Autodesk Fusion 360 part; units mm, degrees
note: some values were not read from the file. Set by a fixed rule: which sketch regions a step uses.
(part 52 of 59)
  spline S32 degree 5 poles (-9.8472, -14.8251) (-9.8472, -14.8252) (-9.8473, -14.8254) (-9.8474, -14.8257) (-9.8475, -14.8262) (-9.8478, -14.8269) (-9.8481, -14.8277) (-9.8484, -14.8286) (-9.8487, -14.8296) (-9.8491, -14.8308) (-9.8495, -14.832) (-9.85, -14.8334) (-9.8505, -14.8348) (-9.851, -14.8364) (-9.8515, -14.838) (-9.8521, -14.8398) (-9.8527, -14.8416) (-9.8533, -14.8435) (-9.8539, -14.8456) (-9.8546, -14.8477) (-9.8553, -14.8499) (-9.856, -14.8523) (-9.8568, -14.8547) (-9.8575, -14.8572) (-9.8583, -14.8598) (-9.8591, -14.8625) (-9.86, -14.8652) (-9.8608, -14.8681) (-9.8617, -14.871) (-9.8626, -14.8741) (-9.8635, -14.8772) (-9.8645, -14.8804) (-9.8654, -14.8837) (-9.8664, -14.887) (-9.8674, -14.8905) (-9.8684, -14.894) (-9.8694, -14.8976) (-9.8704, -14.9013) (-9.8715, -14.9051) (-9.8725, -14.909) (-9.8736, -14.9129) (-9.8747, -14.9169) (-9.8758, -14.921) (-9.8769, -14.9252) (-9.878, -14.9294) (-9.8792, -14.9337) (-9.8803, -14.9381) (-9.8815, -14.9426) (-9.8827, -14.9471) (-9.8838, -14.9517) (-9.885, -14.9564) (-9.8862, -14.9612) (-9.8874, -14.966) (-9.8887, -14.9709) (-9.8899, -14.9759) (-9.8911, -14.981) (-9.8924, -14.9861) (-9.8936, -14.9912) (-9.8949, -14.9965) (-9.8962, -15.0018) (-9.8974, -15.0072) (-9.8987, -15.0127) (-9.9, -15.0182) (-9.9013, -15.0238) (-9.9026, -15.0294) (-9.9039, -15.0352) (-9.9052, -15.0409) (-9.9065, -15.0468) (-9.9079, -15.0527) (-9.9092, -15.0587) (-9.9105, -15.0647) (-9.9118, -15.0709) (-9.9132, -15.077) (-9.9145, -15.0833) (-9.9158, -15.0896) (-9.9172, -15.0959) (-9.9185, -15.1023) (-9.9199, -15.1088) (-9.9212, -15.1154) (-9.9225, -15.122) (-9.9239, -15.1286) (-9.9252, -15.1353) (-9.9266, -15.1421) (-9.9279, -15.149) (-9.9293, -15.1559) (-9.9306, -15.1628) (-9.932, -15.1698) (-9.9333, -15.1769) (-9.9347, -15.1841) (-9.936, -15.1912) (-9.9374, -15.1985) (-9.9387, -15.2058) (-9.9401, -15.2132) (-9.9414, -15.2206) (-9.9428, -15.228) (-9.9441, -15.2356) (-9.9454, -15.2431) (-9.9468, -15.2508) (-9.9481, -15.2585) (-9.9494, -15.2662) (-9.9508, -15.274) (-9.9521, -15.2819) (-9.9534, -15.2898) (-9.9547, -15.2977) (-9.956, -15.3057) (-9.9573, -15.3138) (-9.9586, -15.3219) (-9.9599, -15.3301) (-9.9612, -15.3383) (-9.9625, -15.3466) (-9.9638, -15.3549) (-9.9651, -15.3633) (-9.9664, -15.3717) (-9.9676, -15.3802) (-9.9689, -15.3887) (-9.9701, -15.3973) (-9.9714, -15.4059) (-9.9726, -15.4146) (-9.9739, -15.4233) (-9.9751, -15.4321) (-9.9763, -15.4409) (-9.9776, -15.4498) (-9.9788, -15.4587) (-9.98, -15.4677) (-9.9812, -15.4767) (-9.9824, -15.4858) (-9.9836, -15.4949) (-9.9847, -15.504) (-9.9859, -15.5133) (-9.9871, -15.5225) (-9.9882, -15.5318) (-9.9894, -15.5412) (-9.9905, -15.5506) (-9.9916, -15.56) (-9.9928, -15.5695) (-9.9939, -15.579) (-9.995, -15.5886) (-9.9961, -15.5982) (-9.9972, -15.6079) (-9.9983, -15.6176) (-9.9993, -15.6274) (-10.0004, -15.6372) (-10.0014, -15.647) (-10.0025, -15.6569) (-10.0035, -15.6668) (-10.0045, -15.6768) (-10.0055, -15.6868) (-10.0065, -15.6969) (-10.0075, -15.707) (-10.0085, -15.7172) (-10.0095, -15.7274) (-10.0104, -15.7376) (-10.0114, -15.7479) (-10.0123, -15.7582) (-10.0133, -15.7686) (-10.0142, -15.779) (-10.0151, -15.7894) (-10.016, -15.7999) (-10.0169, -15.8105) (-10.0177, -15.821) (-10.0186, -15.8317) (-10.0195, -15.8423) (-10.0203, -15.853) (-10.0211, -15.8638) (-10.0219, -15.8745) (-10.0227, -15.8854) (-10.0235, -15.8962) (-10.0243, -15.9071) (-10.0251, -15.9181) (-10.0258, -15.929) (-10.0266, -15.94) (-10.0273, -15.9511) (-10.028, -15.9622) (-10.0287, -15.9733) (-10.0294, -15.9845) (-10.0301, -15.9957) (-10.0308, -16.007) (-10.0314, -16.0183) (-10.0321, -16.0296) (-10.0327, -16.041) (-10.0333, -16.0524) (-10.0339, -16.0638) (-10.0345, -16.0753) (-10.0351, -16.0868) (-10.0356, -16.0984) (-10.0362, -16.11) (-10.0367, -16.1216) (-10.0372, -16.1333) (-10.0377, -16.145) (-10.0382, -16.1567) (-10.0387, -16.1685) (-10.0392, -16.1803) (-10.0396, -16.1922) (-10.04, -16.2041) (-10.0405, -16.216) (-10.0409, -16.228) (-10.0412, -16.24) (-10.0416, -16.252) (-10.042, -16.2641) (-10.0423, -16.2762) (-10.0427, -16.2883) (-10.043, -16.3005) (-10.0433, -16.3127) (-10.0436, -16.3249) (-10.0438, -16.3372) (-10.0441, -16.3495) (-10.0443, -16.3619) (-10.0445, -16.3743) (-10.0448, -16.3867) (-10.0449, -16.3991) (-10.0451, -16.4116) (-10.0453, -16.4241) (-10.0454, -16.4367) (-10.0456, -16.4493) (-10.0457, -16.4619) (-10.0458, -16.4745) (-10.0458, -16.4872) (-10.0459, -16.5) (-10.046, -16.5127) (-10.046, -16.5255) (-10.046, -16.5383) (-10.046, -16.5512) (-10.046, -16.5641) (-10.046, -16.577) (-10.0459, -16.5899) (-10.0458, -16.6029) (-10.0458, -16.6159) (-10.0457, -16.629) (-10.0455, -16.642) (-10.0454, -16.6551) (-10.0453, -16.6683) (-10.0451, -16.6815) (-10.0449, -16.6947) (-10.0447, -16.7079) (-10.0445, -16.7212) (-10.0442, -16.7345) (-10.044, -16.7478) (-10.0437, -16.7612) (-10.0434, -16.7745) (-10.0431, -16.788) (-10.0428, -16.8014) (-10.0425, -16.8122) (-10.0423, -16.8203) (-10.0422, -16.8257) (-10.0421, -16.8284) knots 0 0 0 0 0 0 0.00416667 0.00833333 0.0125 0.01666667 0.02083333 0.025 0.02916667 0.03333333 0.0375 0.04166667 0.04583333 0.05 0.05416667 0.05833333 0.0625 0.06666667 0.07083333 0.075 0.07916667 0.08333333 0.0875 0.09166667 0.09583333 0.1 0.10416667 0.10833333 0.1125 0.11666667 0.12083333 0.125 0.12916667 0.13333333 0.1375 0.14166667 0.14583333 0.15 0.15416667 0.15833333 0.1625 0.16666667 0.17083333 0.175 0.17916667 0.18333333 0.1875 0.19166667 0.19583333 0.2 0.20416667 0.20833333 0.2125 0.21666667 0.22083333 0.225 0.22916667 0.23333333 0.2375 0.24166667 0.24583333 0.25 0.25416667 0.25833333 0.2625 0.26666667 0.27083333 0.275 0.27916667 0.28333333 0.2875 0.29166667 0.29583333 0.3 0.30416667 0.30833333 0.3125 0.31666667 0.32083333 0.325 0.32916667 0.33333333 0.3375 0.34166667 0.34583333 0.35 0.35416667 0.35833333 0.3625 0.36666667 0.37083333 0.375 0.37916667 0.38333333 0.3875 0.39166667 0.39583333 0.4 0.40416667 0.40833333 0.4125 0.41666667 0.42083333 0.425 0.42916667 0.43333333 0.4375 0.44166667 0.44583333 0.45 0.45416667 0.45833333 0.4625 0.46666667 0.47083333 0.475 0.47916667 0.48333333 0.4875 0.49166667 0.49583333 0.5 0.50416667 0.50833333 0.5125 0.51666667 0.52083333 0.525 0.52916667 0.53333333 0.5375 0.54166667 0.54583333 0.55 0.55416667 0.55833333 0.5625 0.56666667 0.57083333 0.575 0.57916667 0.58333333 0.5875 0.59166667 0.59583333 0.6 0.60416667 0.60833333 0.6125 0.61666667 0.62083333 0.625 0.62916667 0.63333333 0.6375 0.64166667 0.64583333 0.65 0.65416667 0.65833333 0.6625 0.66666667 0.67083333 0.675 0.67916667 0.68333333 0.6875 0.69166667 0.69583333 0.7 0.70416667 0.70833333 0.7125 0.71666667 0.72083333 0.725 0.72916667 0.73333333 0.7375 0.74166667 0.74583333 0.75 0.75416667 0.75833333 0.7625 0.76666667 0.77083333 0.775 0.77916667 0.78333333 0.7875 0.79166667 0.79583333 0.8 0.80416667 0.80833333 0.8125 0.81666667 0.82083333 0.825 0.82916667 0.83333333 0.8375 0.84166667 0.84583333 0.85 0.85416667 0.85833333 0.8625 0.86666667 0.87083333 0.875 0.87916667 0.88333333 0.8875 0.89166667 0.89583333 0.9 0.90416667 0.90833333 0.9125 0.91666667 0.92083333 0.925 0.92916667 0.93333333 0.9375 0.94166667 0.94583333 0.95 0.95416667 0.95833333 0.9625 0.96666667 0.97083333 0.975 0.97916667 0.98333333 0.9875 0.99166667 0.99583333 1 1 1 1 1 1
  arc A33 (-10.0421, -16.8284) -> (-9.1146, -17.1298) centre (0, 12.5) ccw
  spline S33 degree 5 poles (-9.1146, -17.1298) (-9.1129, -17.1276) (-9.1096, -17.1234) (-9.1047, -17.1169) (-9.0981, -17.1084) (-9.09, -17.0977) (-9.0818, -17.087) (-9.0737, -17.0763) (-9.0657, -17.0657) (-9.0576, -17.055) (-9.0496, -17.0444) (-9.0416, -17.0338) (-9.0337, -17.0232) (-9.0258, -17.0127) (-9.0179, -17.0021) (-9.0101, -16.9915) (-9.0022, -16.981) (-8.9945, -16.9705) (-8.9867, -16.96) (-8.979, -16.9495) (-8.9713, -16.9391) (-8.9637, -16.9286) (-8.956, -16.9182) (-8.9485, -16.9078) (-8.9409, -16.8974) (-8.9334, -16.887) (-8.9259, -16.8766) (-8.9184, -16.8663) (-8.911, -16.856) (-8.9036, -16.8457) (-8.8963, -16.8354) (-8.8889, -16.8251) (-8.8816, -16.8148) (-8.8744, -16.8046) (-8.8671, -16.7944) (-8.86, -16.7842) (-8.8528, -16.774) (-8.8457, -16.7638) (-8.8386, -16.7537) (-8.8315, -16.7435) (-8.8245, -16.7334) (-8.8175, -16.7233) (-8.8105, -16.7132) (-8.8036, -16.7032) (-8.7967, -16.6932) (-8.7898, -16.6831) (-8.783, -16.6731) (-8.7762, -16.6632) (-8.7694, -16.6532) (-8.7626, -16.6433) (-8.7559, -16.6334) (-8.7493, -16.6235) (-8.7426, -16.6136) (-8.736, -16.6037) (-8.7295, -16.5939) (-8.7229, -16.5841) (-8.7164, -16.5743) (-8.7099, -16.5646) (-8.7035, -16.5548) (-8.6971, -16.5451) (-8.6907, -16.5354) (-8.6844, -16.5257) (-8.6781, -16.516) (-8.6718, -16.5064) (-8.6656, -16.4968) (-8.6593, -16.4872) (-8.6532, -16.4776) (-8.647, -16.4681) (-8.6409, -16.4586) (-8.6348, -16.4491) (-8.6288, -16.4396) (-8.6228, -16.4302) (-8.6168, -16.4207) (-8.6109, -16.4113) (-8.605, -16.402) (-8.5991, -16.3926) (-8.5932, -16.3833) (-8.5874, -16.374) (-8.5817, -16.3647) (-8.5759, -16.3555) (-8.5702, -16.3462) (-8.5645, -16.337) (-8.5589, -16.3279) (-8.5533, -16.3187) (-8.5477, -16.3096) (-8.5422, -16.3005) (-8.5367, -16.2914) (-8.5312, -16.2824) (-8.5257, -16.2734) (-8.5203, -16.2644) (-8.515, -16.2554) (-8.5096, -16.2465) (-8.5043, -16.2376) (-8.499, -16.2287) (-8.4938, -16.2199) (-8.4886, -16.211) (-8.4834, -16.2022) (-8.4783, -16.1935) (-8.4732, -16.1847) (-8.4681, -16.176) (-8.463, -16.1674) (-8.458, -16.1587) (-8.4531, -16.1501) (-8.4481, -16.1415) (-8.4432, -16.133) (-8.4384, -16.1244) (-8.4335, -16.116) (-8.4287, -16.1075) (-8.4239, -16.0991) (-8.4192, -16.0907) (-8.4145, -16.0823) (-8.4098, -16.074) (-8.4052, -16.0657) (-8.4006, -16.0574) (-8.396, -16.0491) (-8.3915, -16.0409) (-8.387, -16.0328) (-8.3825, -16.0246) (-8.3781, -16.0165) (-8.3737, -16.0085) (-8.3693, -16.0004) (-8.365, -15.9924) (-8.3607, -15.9845) (-8.3565, -15.9765) (-8.3522, -15.9686) (-8.348, -15.9608) (-8.3439, -15.9529) (-8.3398, -15.9452) (-8.3357, -15.9374) (-8.3316, -15.9297) (-8.3276, -15.922) (-8.3236, -15.9144) (-8.3196, -15.9068) (-8.3157, -15.8992) (-8.3118, -15.8917) (-8.308, -15.8842) (-8.3042, -15.8767) (-8.3004, -15.8693) (-8.2966, -15.8619) (-8.2929, -15.8546) (-8.2892, -15.8473) (-8.2856, -15.8401) (-8.282, -15.8329) (-8.2784, -15.8257) (-8.2748, -15.8186) (-8.2713, -15.8115) (-8.2678, -15.8044) (-8.2644, -15.7974) (-8.261, -15.7905) (-8.2576, -15.7835) (-8.2543, -15.7767) (-8.251, -15.7698) (-8.2477, -15.763) (-8.2445, -15.7563) (-8.2412, -15.7496) (-8.2381, -15.7429) (-8.2349, -15.7363) (-8.2318, -15.7298) (-8.2288, -15.7233) (-8.2257, -15.7168) (-8.2227, -15.7104) (-8.2198, -15.704) (-8.2169, -15.6977) (-8.214, -15.6914) (-8.2111, -15.6851) (-8.2083, -15.679) (-8.2055, -15.6728) (-8.2027, -15.6667) (-8.2, -15.6607) (-8.1973, -15.6547) (-8.1947, -15.6488) (-8.192, -15.6429) (-8.1895, -15.6371) (-8.1869, -15.6313) (-8.1844, -15.6256) (-8.1819, -15.6199) (-8.1795, -15.6143) (-8.177, -15.6087) (-8.1747, -15.6032) (-8.1723, -15.5978) (-8.17, -15.5924) (-8.1677, -15.587) (-8.1655, -15.5818) (-8.1633, -15.5765) (-8.1611, -15.5714) (-8.159, -15.5663) (-8.1569, -15.5612) (-8.1548, -15.5562) (-8.1528, -15.5513) (-8.1508, -15.5464) (-8.1488, -15.5416) (-8.1469, -15.5369) (-8.145, -15.5322) (-8.1432, -15.5276) (-8.1413, -15.523) (-8.1395, -15.5185) (-8.1378, -15.5141) (-8.1361, -15.5097) (-8.1344, -15.5054) (-8.1327, -15.5012) (-8.1311, -15.497) (-8.1295, -15.4929) (-8.128, -15.4889) (-8.1265, -15.4849) (-8.125, -15.4811) (-8.1236, -15.4772) (-8.1222, -15.4735) (-8.1208, -15.4698) (-8.1194, -15.4662) (-8.1181, -15.4627) (-8.1169, -15.4593) (-8.1156, -15.4559) (-8.1144, -15.4526) (-8.1133, -15.4494) (-8.1121, -15.4462) (-8.1111, -15.4432) (-8.11, -15.4402) (-8.109, -15.4373) (-8.108, -15.4345) (-8.107, -15.4318) (-8.1061, -15.4291) (-8.1052, -15.4265) (-8.1044, -15.4241) (-8.1036, -15.4217) (-8.1028, -15.4194) (-8.102, -15.4172) (-8.1013, -15.415) (-8.1007, -15.413) (-8.1, -15.4111) (-8.0994, -15.4092) (-8.0988, -15.4075) (-8.0983, -15.4058) (-8.0978, -15.4043) (-8.0973, -15.4028) (-8.0969, -15.4015) (-8.0965, -15.4002) (-8.0962, -15.3991) (-8.0958, -15.398) (-8.0956, -15.3971) (-8.0953, -15.3963) (-8.0951, -15.3956) (-8.0949, -15.3951) (-8.0948, -15.3948) (-8.0948, -15.3946) (-8.0948, -15.3945) knots -1 -1 -1 -1 -1 -1 -0.99583333 -0.99166667 -0.9875 -0.98333333 -0.97916667 -0.975 -0.97083333 -0.96666667 -0.9625 -0.95833333 -0.95416667 -0.95 -0.94583333 -0.94166667 -0.9375 -0.93333333 -0.92916667 -0.925 -0.92083333 -0.91666667 -0.9125 -0.90833333 -0.90416667 -0.9 -0.89583333 -0.89166667 -0.8875 -0.88333333 -0.87916667 -0.875 -0.87083333 -0.86666667 -0.8625 -0.85833333 -0.85416667 -0.85 -0.84583333 -0.84166667 -0.8375 -0.83333333 -0.82916667 -0.825 -0.82083333 -0.81666667 -0.8125 -0.80833333 -0.80416667 -0.8 -0.79583333 -0.79166667 -0.7875 -0.78333333 -0.77916667 -0.775 -0.77083333 -0.76666667 -0.7625 -0.75833333 -0.75416667 -0.75 -0.74583333 -0.74166667 -0.7375 -0.73333333 -0.72916667 -0.725 -0.72083333 -0.71666667 -0.7125 -0.70833333 -0.70416667 -0.7 -0.69583333 -0.69166667 -0.6875 -0.68333333 -0.67916667 -0.675 -0.67083333 -0.66666667 -0.6625 -0.65833333 -0.65416667 -0.65 -0.64583333 -0.64166667 -0.6375 -0.63333333 -0.62916667 -0.625 -0.62083333 -0.61666667 -0.6125 -0.60833333 -0.60416667 -0.6 -0.59583333 -0.59166667 -0.5875 -0.58333333 -0.57916667 -0.575 -0.57083333 -0.56666667 -0.5625 -0.55833333 -0.55416667 -0.55 -0.54583333 -0.54166667 -0.5375 -0.53333333 -0.52916667 -0.525 -0.52083333 -0.51666667 -0.5125 -0.50833333 -0.50416667 -0.5 -0.49583333 -0.49166667 -0.4875 -0.48333333 -0.47916667 -0.475 -0.47083333 -0.46666667 -0.4625 -0.45833333 -0.45416667 -0.45 -0.44583333 -0.44166667 -0.4375 -0.43333333 -0.42916667 -0.425 -0.42083333 -0.41666667 -0.4125 -0.40833333 -0.40416667 -0.4 -0.39583333 -0.39166667 -0.3875 -0.38333333 -0.37916667 -0.375 -0.37083333 -0.36666667 -0.3625 -0.35833333 -0.35416667 -0.35 -0.34583333 -0.34166667 -0.3375 -0.33333333 -0.32916667 -0.325 -0.32083333 -0.31666667 -0.3125 -0.30833333 -0.30416667 -0.3 -0.29583333 -0.29166667 -0.2875 -0.28333333 -0.27916667 -0.275 -0.27083333 -0.26666667 -0.2625 -0.25833333 -0.25416667 -0.25 -0.24583333 -0.24166667 -0.2375 -0.23333333 -0.22916667 -0.225 -0.22083333 -0.21666667 -0.2125 -0.20833333 -0.20416667 -0.2 -0.19583333 -0.19166667 -0.1875 -0.18333333 -0.17916667 -0.175 -0.17083333 -0.16666667 -0.1625 -0.15833333 -0.15416667 -0.15 -0.14583333 -0.14166667 -0.1375 -0.13333333 -0.12916667 -0.125 -0.12083333 -0.11666667 -0.1125 -0.10833333 -0.10416667 -0.1 -0.09583333 -0.09166667 -0.0875 -0.08333333 -0.07916667 -0.075 -0.07083333 -0.06666667 -0.0625 -0.05833333 -0.05416667 -0.05 -0.04583333 -0.04166667 -0.0375 -0.03333333 -0.02916667 -0.025 -0.02083333 -0.01666667 -0.0125 -0.00833333 -0.00416667 0 0 0 0 0 0
  line L67 (-8.0948, -15.3945) -> (-8.0945, -15.3937)
  line L68 (-8.0945, -15.3937) -> (-8.0125, -15.1109)
  arc A34 (-8.0125, -15.1109) -> (-6.8665, -15.418) centre (0, 12.5) ccw
  line L69 (-6.8665, -15.418) -> (-6.9368, -15.7039)
  line L70 (-6.9368, -15.7039) -> (-6.937, -15.7047)
  spline S34 degree 5 poles (-6.937, -15.7047) (-6.937, -15.7048) (-6.937, -15.705) (-6.9371, -15.7053) (-6.9372, -15.7058) (-6.9374, -15.7065) (-6.9376, -15.7074) (-6.9378, -15.7083) (-6.9381, -15.7094) (-6.9383, -15.7106) (-6.9386, -15.7118) (-6.9389, -15.7132) (-6.9392, -15.7147) (-6.9396, -15.7163) (-6.9399, -15.718) (-6.9403, -15.7198) (-6.9407, -15.7217) (-6.9411, -15.7237) (-6.9416, -15.7258) (-6.942, -15.728) (-6.9425, -15.7303) (-6.9429, -15.7327) (-6.9434, -15.7351) (-6.9439, -15.7377) (-6.9445, -15.7404) (-6.945, -15.7431) (-6.9455, -15.746) (-6.9461, -15.7489) (-6.9466, -15.7519) (-6.9472, -15.755) (-6.9478, -15.7582) (-6.9484, -15.7615) (-6.949, -15.7649) (-6.9496, -15.7683) (-6.9502, -15.7719) (-6.9508, -15.7755) (-6.9515, -15.7792) (-6.9521, -15.783) (-6.9528, -15.7868) (-6.9534, -15.7908) (-6.9541, -15.7948) (-6.9547, -15.7989) (-6.9554, -15.8031) (-6.9561, -15.8074) (-6.9568, -15.8117) (-6.9574, -15.8161) (-6.9581, -15.8206) (-6.9588, -15.8252) (-6.9595, -15.8298) (-6.9602, -15.8345) (-6.9609, -15.8393) (-6.9616, -15.8442) (-6.9623, -15.8491) (-6.963, -15.8541) (-6.9637, -15.8592) (-6.9644, -15.8643) (-6.9651, -15.8695) (-6.9658, -15.8748) (-6.9665, -15.8802) (-6.9672, -15.8856) (-6.9679, -15.8911) (-6.9686, -15.8966) (-6.9693, -15.9023) (-6.97, -15.908) (-6.9707, -15.9137) (-6.9714, -15.9196) (-6.9721, -15.9255) (-6.9728, -15.9314) (-6.9735, -15.9374) (-6.9742, -15.9435) (-6.9749, -15.9497) (-6.9756, -15.9559) (-6.9763, -15.9622) (-6.9769, -15.9685) (-6.9776, -15.9749) (-6.9783, -15.9814) (-6.9789, -15.9879) (-6.9796, -15.9945) (-6.9803, -16.0011) (-6.9809, -16.0078) (-6.9816, -16.0146) (-6.9822, -16.0214) (-6.9828, -16.0283) (-6.9835, -16.0353) (-6.9841, -16.0423) (-6.9847, -16.0493) (-6.9853, -16.0564) (-6.9859, -16.0636) (-6.9865, -16.0709) (-6.9871, -16.0781) (-6.9877, -16.0855) (-6.9882, -16.0929) (-6.9888, -16.1004) (-6.9894, -16.1079) (-6.9899, -16.1154) (-6.9905, -16.1231) (-6.991, -16.1307) (-6.9915, -16.1385) (-6.9921, -16.1463) (-6.9926, -16.1541) (-6.9931, -16.162) (-6.9936, -16.17) (-6.994, -16.178) (-6.9945, -16.186) (-6.995, -16.1941) (-6.9954, -16.2023) (-6.9959, -16.2105) (-6.9963, -16.2187) (-6.9968, -16.227) (-6.9972, -16.2354) (-6.9976, -16.2438) (-6.998, -16.2523) (-6.9984, -16.2608) (-6.9987, -16.2694) (-6.9991, -16.278) (-6.9995, -16.2866) (-6.9998, -16.2953) (-7.0001, -16.3041) (-7.0005, -16.3129) (-7.0008, -16.3218) (-7.0011, -16.3307) (-7.0014, -16.3396) (-7.0016, -16.3486) (-7.0019, -16.3577) (-7.0021, -16.3668) (-7.0024, -16.3759) (-7.0026, -16.3851) (-7.0028, -16.3943) (-7.003, -16.4036) (-7.0032, -16.4129) (-7.0034, -16.4223) (-7.0036, -16.4317) (-7.0037, -16.4412) (-7.0038, -16.4507) (-7.004, -16.4602) (-7.0041, -16.4698) (-7.0042, -16.4795) (-7.0043, -16.4892) (-7.0043, -16.4989) (-7.0044, -16.5087) (-7.0044, -16.5185) (-7.0045, -16.5284) (-7.0045, -16.5383) (-7.0045, -16.5482) (-7.0045, -16.5582) (-7.0044, -16.5682) (-7.0044, -16.5783) (-7.0043, -16.5884) (-7.0043, -16.5986) (-7.0042, -16.6088) (-7.0041, -16.619) (-7.004, -16.6293) (-7.0038, -16.6396) (-7.0037, -16.65) (-7.0035, -16.6604) (-7.0034, -16.6708) (-7.0032, -16.6813) (-7.003, -16.6919) (-7.0028, -16.7024) (-7.0025, -16.713) (-7.0023, -16.7237) (-7.002, -16.7344) (-7.0017, -16.7451) (-7.0014, -16.7559) (-7.0011, -16.7667) (-7.0008, -16.7775) (-7.0004, -16.7884) (-7.0001, -16.7993) (-6.9997, -16.8103) (-6.9993, -16.8213) (-6.9989, -16.8323) (-6.9984, -16.8434) (-6.998, -16.8545) (-6.9975, -16.8657) (-6.997, -16.8768) (-6.9965, -16.8881) (-6.996, -16.8993) (-6.9955, -16.9106) (-6.995, -16.922) (-6.9944, -16.9333) (-6.9938, -16.9447) (-6.9932, -16.9562) (-6.9926, -16.9677) (-6.992, -16.9792) (-6.9913, -16.9907) (-6.9906, -17.0023) (-6.99, -17.014) (-6.9892, -17.0256) (-6.9885, -17.0373) (-6.9878, -17.049) (-6.987, -17.0608) (-6.9863, -17.0726) (-6.9855, -17.0844) (-6.9846, -17.0963) (-6.9838, -17.1082) (-6.983, -17.1201) (-6.9821, -17.1321) (-6.9812, -17.1441) (-6.9803, -17.1562) (-6.9794, -17.1682) (-6.9784, -17.1803) (-6.9775, -17.1925) (-6.9765, -17.2047) (-6.9755, -17.2169) (-6.9745, -17.2291) (-6.9735, -17.2414) (-6.9724, -17.2537) (-6.9713, -17.266) (-6.9702, -17.2784) (-6.9691, -17.2908) (-6.968, -17.3032) (-6.9669, -17.3157) (-6.9657, -17.3282) (-6.9645, -17.3407) (-6.9633, -17.3533) (-6.9621, -17.3659) (-6.9608, -17.3785) (-6.9596, -17.3912) (-6.9583, -17.4039) (-6.957, -17.4166) (-6.9556, -17.4293) (-6.9543, -17.4421) (-6.9529, -17.4549) (-6.9516, -17.4678) (-6.9501, -17.4806) (-6.9487, -17.4935) (-6.9473, -17.5065) (-6.9458, -17.5194) (-6.9443, -17.5324) (-6.9428, -17.5455) (-6.9413, -17.5585) (-6.9398, -17.5716) (-6.9382, -17.5847) (-6.9366, -17.5979) (-6.935, -17.611) (-6.9334, -17.6242) (-6.9317, -17.6375) (-6.9301, -17.6507) (-6.9284, -17.664) (-6.9267, -17.6773) (-6.925, -17.6907) (-6.9236, -17.7014) (-6.9225, -17.7094) (-6.9218, -17.7148) (-6.9214, -17.7174) knots 0 0 0 0 0 0 0.00416667 0.00833333 0.0125 0.01666667 0.02083333 0.025 0.02916667 0.03333333 0.0375 0.04166667 0.04583333 0.05 0.05416667 0.05833333 0.0625 0.06666667 0.07083333 0.075 0.07916667 0.08333333 0.0875 0.09166667 0.09583333 0.1 0.10416667 0.10833333 0.1125 0.11666667 0.12083333 0.125 0.12916667 0.13333333 0.1375 0.14166667 0.14583333 0.15 0.15416667 0.15833333 0.1625 0.16666667 0.17083333 0.175 0.17916667 0.18333333 0.1875 0.19166667 0.19583333 0.2 0.20416667 0.20833333 0.2125 0.21666667 0.22083333 0.225 0.22916667 0.23333333 0.2375 0.24166667 0.24583333 0.25 0.25416667 0.25833333 0.2625 0.26666667 0.27083333 0.275 0.27916667 0.28333333 0.2875 0.29166667 0.29583333 0.3 0.30416667 0.30833333 0.3125 0.31666667 0.32083333 0.325 0.32916667 0.33333333 0.3375 0.34166667 0.34583333 0.35 0.35416667 0.35833333 0.3625 0.36666667 0.37083333 0.375 0.37916667 0.38333333 0.3875 0.39166667 0.39583333 0.4 0.40416667 0.40833333 0.4125 0.41666667 0.42083333 0.425 0.42916667 0.43333333 0.4375 0.44166667 0.44583333 0.45 0.45416667 0.45833333 0.4625 0.46666667 0.47083333 0.475 0.47916667 0.48333333 0.4875 0.49166667 0.49583333 0.5 0.50416667 0.50833333 0.5125 0.51666667 0.52083333 0.525 0.52916667 0.53333333 0.5375 0.54166667 0.54583333 0.55 0.55416667 0.55833333 0.5625 0.56666667 0.57083333 0.575 0.57916667 0.58333333 0.5875 0.59166667 0.59583333 0.6 0.60416667 0.60833333 0.6125 0.61666667 0.62083333 0.625 0.62916667 0.63333333 0.6375 0.64166667 0.64583333 0.65 0.65416667 0.65833333 0.6625 0.66666667 0.67083333 0.675 0.67916667 0.68333333 0.6875 0.69166667 0.69583333 0.7 0.70416667 0.70833333 0.7125 0.71666667 0.72083333 0.725 0.72916667 0.73333333 0.7375 0.74166667 0.74583333 0.75 0.75416667 0.75833333 0.7625 0.76666667 0.77083333 0.775 0.77916667 0.78333333 0.7875 0.79166667 0.79583333 0.8 0.80416667 0.80833333 0.8125 0.81666667 0.82083333 0.825 0.82916667 0.83333333 0.8375 0.84166667 0.84583333 0.85 0.85416667 0.85833333 0.8625 0.86666667 0.87083333 0.875 0.87916667 0.88333333 0.8875 0.89166667 0.89583333 0.9 0.90416667 0.90833333 0.9125 0.91666667 0.92083333 0.925 0.92916667 0.93333333 0.9375 0.94166667 0.94583333 0.95 0.95416667 0.95833333 0.9625 0.96666667 0.97083333 0.975 0.97916667 0.98333333 0.9875 0.99166667 0.99583333 1 1 1 1 1 1
  arc A35 (-6.9214, -17.7174) -> (-5.9675, -17.9202) centre (0, 12.5) ccw
  spline S35 degree 5 poles (-5.9675, -17.9202) (-5.9661, -17.9179) (-5.9633, -17.9133) (-5.959, -17.9064) (-5.9534, -17.8972) (-5.9464, -17.8857) (-5.9394, -17.8742) (-5.9325, -17.8628) (-5.9255, -17.8513) (-5.9187, -17.8399) (-5.9118, -17.8285) (-5.905, -17.8171) (-5.8982, -17.8058) (-5.8914, -17.7944) (-5.8847, -17.7831) (-5.878, -17.7718) (-5.8713, -17.7605) (-5.8647, -17.7492) (-5.8581, -17.738) (-5.8515, -17.7268) (-5.8449, -17.7156) (-5.8384, -17.7044) (-5.8319, -17.6932) (-5.8255, -17.6821) (-5.8191, -17.6709) (-5.8127, -17.6598) (-5.8063, -17.6487) (-5.8, -17.6377) (-5.7937, -17.6266) (-5.7874, -17.6156) (-5.7811, -17.6046) (-5.7749, -17.5936) (-5.7688, -17.5826) (-5.7626, -17.5717) (-5.7565, -17.5608) (-5.7504, -17.5499) (-5.7443, -17.539) (-5.7383, -17.5281) (-5.7323, -17.5173) (-5.7263, -17.5065) (-5.7204, -17.4957) (-5.7145, -17.4849) (-5.7086, -17.4742) (-5.7028, -17.4634) (-5.697, -17.4527) (-5.6912, -17.4421) (-5.6854, -17.4314) (-5.6797, -17.4208) (-5.674, -17.4102) (-5.6683, -17.3996) (-5.6627, -17.389) (-5.6571, -17.3785) (-5.6515, -17.368) (-5.646, -17.3575) (-5.6405, -17.347) (-5.635, -17.3366) (-5.6296, -17.3262) (-5.6242, -17.3158) (-5.6188, -17.3054) (-5.6134, -17.2951) (-5.6081, -17.2847) (-5.6028, -17.2745) (-5.5975, -17.2642) (-5.5923, -17.254) (-5.5871, -17.2437) (-5.5819, -17.2336) (-5.5768, -17.2234) (-5.5717, -17.2133) (-5.5666, -17.2032) (-5.5615, -17.1931) (-5.5565, -17.183) (-5.5515, -17.173) (-5.5466, -17.163) (-5.5416, -17.153) (-5.5367, -17.1431) (-5.5319, -17.1332) (-5.527, -17.1233) (-5.5222, -17.1134) (-5.5175, -17.1036) (-5.5127, -17.0938) (-5.508, -17.084) (-5.5033, -17.0743) (-5.4987, -17.0646) (-5.494, -17.0549) (-5.4895, -17.0452) (-5.4849, -17.0356) (-5.4804, -17.026) (-5.4759, -17.0165) (-5.4714, -17.0069) (-5.467, -16.9974) (-5.4625, -16.9879) (-5.4582, -16.9785) (-5.4538, -16.9691) (-5.4495, -16.9597) (-5.4452, -16.9504) (-5.441, -16.941) (-5.4367, -16.9318) (-5.4325, -16.9225) (-5.4284, -16.9133) (-5.4242, -16.9041) (-5.4201, -16.895) (-5.4161, -16.8858) (-5.412, -16.8767) (-5.408, -16.8677) (-5.404, -16.8587) (-5.4001, -16.8497) (-5.3961, -16.8407) (-5.3922, -16.8318) (-5.3884, -16.8229) (-5.3846, -16.8141) (-5.3807, -16.8053) (-5.377, -16.7965) (-5.3732, -16.7878) (-5.3695, -16.779) (-5.3658, -16.7704) (-5.3622, -16.7617) (-5.3586, -16.7531) (-5.355, -16.7446) (-5.3514, -16.7361) (-5.3479, -16.7276) (-5.3444, -16.7191) (-5.3409, -16.7107) (-5.3375, -16.7023) (-5.3341, -16.694) (-5.3307, -16.6857) (-5.3273, -16.6775) (-5.324, -16.6692) (-5.3207, -16.6611) (-5.3175, -16.6529) (-5.3143, -16.6448) (-5.3111, -16.6368) (-5.3079, -16.6288) (-5.3047, -16.6208) (-5.3016, -16.6129) (-5.2986, -16.605) (-5.2955, -16.5971) (-5.2925, -16.5893) (-5.2895, -16.5815) (-5.2865, -16.5738) (-5.2836, -16.5661) (-5.2807, -16.5585) (-5.2778, -16.5509) (-5.275, -16.5433) (-5.2722, -16.5358) (-5.2694, -16.5284) (-5.2666, -16.521) (-5.2639, -16.5136) (-5.2612, -16.5063) (-5.2586, -16.499) (-5.2559, -16.4918) (-5.2533, -16.4846) (-5.2508, -16.4774) (-5.2482, -16.4703) (-5.2457, -16.4633) (-5.2432, -16.4563) (-5.2408, -16.4493) (-5.2383, -16.4424) (-5.2359, -16.4356) (-5.2336, -16.4288) (-5.2312, -16.422) (-5.2289, -16.4153) (-5.2266, -16.4087) (-5.2244, -16.4021) (-5.2222, -16.3955) (-5.22, -16.389) (-5.2178, -16.3826) (-5.2157, -16.3762) (-5.2136, -16.3699) (-5.2115, -16.3636) (-5.2094, -16.3573) (-5.2074, -16.3512) (-5.2054, -16.3451) (-5.2035, -16.339) (-5.2015, -16.333) (-5.1996, -16.327) (-5.1978, -16.3211) (-5.1959, -16.3153) (-5.1941, -16.3095) (-5.1923, -16.3038) (-5.1905, -16.2981) (-5.1888, -16.2925) (-5.1871, -16.2869) (-5.1854, -16.2815) (-5.1838, -16.276) (-5.1822, -16.2707) (-5.1806, -16.2654) (-5.179, -16.2601) (-5.1775, -16.2549) (-5.176, -16.2498) (-5.1745, -16.2448) (-5.173, -16.2398) (-5.1716, -16.2349) (-5.1702, -16.23) (-5.1689, -16.2252) (-5.1675, -16.2205) (-5.1662, -16.2158) (-5.1649, -16.2112) (-5.1637, -16.2067) (-5.1625, -16.2023) (-5.1613, -16.1979) (-5.1601, -16.1936) (-5.1589, -16.1893) (-5.1578, -16.1852) (-5.1567, -16.1811) (-5.1557, -16.1771) (-5.1546, -16.1731) (-5.1536, -16.1693) (-5.1527, -16.1655) (-5.1517, -16.1617) (-5.1508, -16.1581) (-5.1499, -16.1545) (-5.149, -16.1511) (-5.1481, -16.1477) (-5.1473, -16.1443) (-5.1465, -16.1411) (-5.1458, -16.1379) (-5.145, -16.1349) (-5.1443, -16.1319) (-5.1436, -16.129) (-5.143, -16.1262) (-5.1423, -16.1234) (-5.1417, -16.1208) (-5.1411, -16.1182) (-5.1406, -16.1158) (-5.14, -16.1134) (-5.1395, -16.1111) (-5.139, -16.1089) (-5.1386, -16.1069) (-5.1381, -16.1049) (-5.1377, -16.103) (-5.1374, -16.1012) (-5.137, -16.0995) (-5.1367, -16.0979) (-5.1363, -16.0964) (-5.1361, -16.095) (-5.1358, -16.0937) (-5.1356, -16.0925) (-5.1354, -16.0915) (-5.1352, -16.0905) (-5.135, -16.0896) (-5.1349, -16.0889) (-5.1348, -16.0884) (-5.1347, -16.0881) (-5.1347, -16.0879) (-5.1346, -16.0878) knots -1 -1 -1 -1 -1 -1 -0.99583333 -0.99166667 -0.9875 -0.98333333 -0.97916667 -0.975 -0.97083333 -0.96666667 -0.9625 -0.95833333 -0.95416667 -0.95 -0.94583333 -0.94166667 -0.9375 -0.93333333 -0.92916667 -0.925 -0.92083333 -0.91666667 -0.9125 -0.90833333 -0.90416667 -0.9 -0.89583333 -0.89166667 -0.8875 -0.88333333 -0.87916667 -0.875 -0.87083333 -0.86666667 -0.8625 -0.85833333 -0.85416667 -0.85 -0.84583333 -0.84166667 -0.8375 -0.83333333 -0.82916667 -0.825 -0.82083333 -0.81666667 -0.8125 -0.80833333 -0.80416667 -0.8 -0.79583333 -0.79166667 -0.7875 -0.78333333 -0.77916667 -0.775 -0.77083333 -0.76666667 -0.7625 -0.75833333 -0.75416667 -0.75 -0.74583333 -0.74166667 -0.7375 -0.73333333 -0.72916667 -0.725 -0.72083333 -0.71666667 -0.7125 -0.70833333 -0.70416667 -0.7 -0.69583333 -0.69166667 -0.6875 -0.68333333 -0.67916667 -0.675 -0.67083333 -0.66666667 -0.6625 -0.65833333 -0.65416667 -0.65 -0.64583333 -0.64166667 -0.6375 -0.63333333 -0.62916667 -0.625 -0.62083333 -0.61666667 -0.6125 -0.60833333 -0.60416667 -0.6 -0.59583333 -0.59166667 -0.5875 -0.58333333 -0.57916667 -0.575 -0.57083333 -0.56666667 -0.5625 -0.55833333 -0.55416667 -0.55 -0.54583333 -0.54166667 -0.5375 -0.53333333 -0.52916667 -0.525 -0.52083333 -0.51666667 -0.5125 -0.50833333 -0.50416667 -0.5 -0.49583333 -0.49166667 -0.4875 -0.48333333 -0.47916667 -0.475 -0.47083333 -0.46666667 -0.4625 -0.45833333 -0.45416667 -0.45 -0.44583333 -0.44166667 -0.4375 -0.43333333 -0.42916667 -0.425 -0.42083333 -0.41666667 -0.4125 -0.40833333 -0.40416667 -0.4 -0.39583333 -0.39166667 -0.3875 -0.38333333 -0.37916667 -0.375 -0.37083333 -0.36666667 -0.3625 -0.35833333 -0.35416667 -0.35 -0.34583333 -0.34166667 -0.3375 -0.33333333 -0.32916667 -0.325 -0.32083333 -0.31666667 -0.3125 -0.30833333 -0.30416667 -0.3 -0.29583333 -0.29166667 -0.2875 -0.28333333 -0.27916667 -0.275 -0.27083333 -0.26666667 -0.2625 -0.25833333 -0.25416667 -0.25 -0.24583333 -0.24166667 -0.2375 -0.23333333 -0.22916667 -0.225 -0.22083333 -0.21666667 -0.2125 -0.20833333 -0.20416667 -0.2 -0.19583333 -0.19166667 -0.1875 -0.18333333 -0.17916667 -0.175 -0.17083333 -0.16666667 -0.1625 -0.15833333 -0.15416667 -0.15 -0.14583333 -0.14166667 -0.1375 -0.13333333 -0.12916667 -0.125 -0.12083333 -0.11666667 -0.1125 -0.10833333 -0.10416667 -0.1 -0.09583333 -0.09166667 -0.0875 -0.08333333 -0.07916667 -0.075 -0.07083333 -0.06666667 -0.0625 -0.05833333 -0.05416667 -0.05 -0.04583333 -0.04166667 -0.0375 -0.03333333 -0.02916667 -0.025 -0.02083333 -0.01666667 -0.0125 -0.00833333 -0.00416667 0 0 0 0 0 0
  line L71 (-5.1346, -16.0878) -> (-5.1345, -16.087)
  line L72 (-5.1345, -16.087) -> (-5.0824, -15.7972)
  arc A36 (-5.0824, -15.7972) -> (-3.9106, -15.9828) centre (0, 12.5) ccw
  line L73 (-3.9106, -15.9828) -> (-3.9507, -16.2745)
  line L74 (-3.9507, -16.2745) -> (-3.9508, -16.2753)
  spline S36 degree 5 poles (-3.9508, -16.2753) (-3.9508, -16.2754) (-3.9508, -16.2756) (-3.9509, -16.2759) (-3.9509, -16.2764) (-3.951, -16.2772) (-3.9511, -16.278) (-3.9512, -16.279) (-3.9514, -16.2801) (-3.9515, -16.2813) (-3.9517, -16.2826) (-3.9518, -16.284) (-3.952, -16.2855) (-3.9522, -16.2871) (-3.9523, -16.2889) (-3.9525, -16.2907) (-3.9527, -16.2926) (-3.9529, -16.2946) (-3.9531, -16.2968) (-3.9534, -16.299) (-3.9536, -16.3013) (-3.9538, -16.3037) (-3.954, -16.3063) (-3.9543, -16.3089) (-3.9545, -16.3116) (-3.9547, -16.3144) (-3.955, -16.3172) (-3.9552, -16.3202) (-3.9555, -16.3233) (-3.9557, -16.3264) (-3.9559, -16.3297) (-3.9562, -16.333) (-3.9564, -16.3364) (-3.9567, -16.3399) (-3.9569, -16.3435) (-3.9572, -16.3472) (-3.9574, -16.3509) (-3.9577, -16.3547) (-3.9579, -16.3586) (-3.9581, -16.3626) (-3.9584, -16.3667) (-3.9586, -16.3709) (-3.9588, -16.3751) (-3.959, -16.3794) (-3.9593, -16.3838) (-3.9595, -16.3882) (-3.9597, -16.3928) (-3.9599, -16.3974) (-3.9601, -16.4021) (-3.9603, -16.4068) (-3.9605, -16.4117) (-3.9607, -16.4166) (-3.9609, -16.4215) (-3.961, -16.4266) (-3.9612, -16.4317) (-3.9614, -16.4369) (-3.9615, -16.4422) (-3.9617, -16.4475) (-3.9618, -16.4529) (-3.962, -16.4584) (-3.9621, -16.4639) (-3.9622, -16.4695) (-3.9623, -16.4752) (-3.9624, -16.4809) (-3.9625, -16.4867) (-3.9626, -16.4926) (-3.9627, -16.4985) (-3.9627, -16.5045) (-3.9628, -16.5106) (-3.9629, -16.5167) (-3.9629, -16.5229) (-3.9629, -16.5291) (-3.9629, -16.5355) (-3.963, -16.5418) (-3.963, -16.5483) (-3.9629, -16.5548) (-3.9629, -16.5613) (-3.9629, -16.568) (-3.9628, -16.5746) (-3.9628, -16.5814) (-3.9627, -16.5882) (-3.9626, -16.595) (-3.9626, -16.6019) (-3.9625, -16.6089) (-3.9623, -16.6159) (-3.9622, -16.623) (-3.9621, -16.6302) (-3.9619, -16.6374) (-3.9618, -16.6446) (-3.9616, -16.6519) (-3.9614, -16.6593) (-3.9612, -16.6667) (-3.961, -16.6742) (-3.9607, -16.6817) (-3.9605, -16.6893) (-3.9603, -16.697) (-3.96, -16.7047) (-3.9597, -16.7124) (-3.9594, -16.7202) (-3.9591, -16.7281) (-3.9588, -16.736) (-3.9584, -16.7439) (-3.9581, -16.7519) (-3.9577, -16.76) (-3.9573, -16.7681) (-3.9569, -16.7763) (-3.9565, -16.7845) (-3.9561, -16.7927) (-3.9556, -16.801) (-3.9552, -16.8094) (-3.9547, -16.8178) (-3.9542, -16.8263) (-3.9537, -16.8348) (-3.9532, -16.8433) (-3.9526, -16.8519) (-3.9521, -16.8606) (-3.9515, -16.8693) (-3.9509, -16.878) (-3.9503, -16.8868) (-3.9497, -16.8957) (-3.9491, -16.9045) (-3.9484, -16.9135) (-3.9478, -16.9225) (-3.9471, -16.9315) (-3.9464, -16.9406) (-3.9457, -16.9497) (-3.9449, -16.9588) (-3.9442, -16.968) (-3.9434, -16.9773) (-3.9426, -16.9866) (-3.9418, -16.9959) (-3.941, -17.0053) (-3.9402, -17.0147) (-3.9393, -17.0242) (-3.9384, -17.0337) (-3.9375, -17.0433) (-3.9366, -17.0529) (-3.9357, -17.0625) (-3.9348, -17.0722) (-3.9338, -17.0819) (-3.9328, -17.0917) (-3.9318, -17.1015) (-3.9308, -17.1113) (-3.9297, -17.1212) (-3.9287, -17.1312) (-3.9276, -17.1411) (-3.9265, -17.1512) (-3.9254, -17.1612) (-3.9243, -17.1713) (-3.9231, -17.1814) (-3.922, -17.1916) (-3.9208, -17.2018) (-3.9196, -17.2121) (-3.9183, -17.2224) (-3.9171, -17.2327) (-3.9158, -17.2431) (-3.9145, -17.2535) (-3.9132, -17.264) (-3.9119, -17.2744) (-3.9106, -17.285) (-3.9092, -17.2955) (-3.9078, -17.3061) (-3.9064, -17.3168) (-3.905, -17.3274) (-3.9035, -17.3382) (-3.9021, -17.3489) (-3.9006, -17.3597) (-3.8991, -17.3705) (-3.8976, -17.3814) (-3.896, -17.3923) (-3.8945, -17.4032) (-3.8929, -17.4142) (-3.8913, -17.4252) (-3.8896, -17.4362) (-3.888, -17.4473) (-3.8863, -17.4584) (-3.8846, -17.4696) (-3.8829, -17.4807) (-3.8812, -17.492) (-3.8795, -17.5032) (-3.8777, -17.5145) (-3.8759, -17.5258) (-3.8741, -17.5372) (-3.8722, -17.5486) (-3.8704, -17.56) (-3.8685, -17.5714) (-3.8666, -17.5829) (-3.8647, -17.5944) (-3.8628, -17.606) (-3.8608, -17.6176) (-3.8588, -17.6292) (-3.8568, -17.6409) (-3.8548, -17.6525) (-3.8527, -17.6643) (-3.8507, -17.676) (-3.8486, -17.6878) (-3.8464, -17.6996) (-3.8443, -17.7115) (-3.8422, -17.7233) (-3.84, -17.7353) (-3.8378, -17.7472) (-3.8356, -17.7592) (-3.8333, -17.7712) (-3.831, -17.7832) (-3.8288, -17.7953) (-3.8264, -17.8074) (-3.8241, -17.8195) (-3.8217, -17.8317) (-3.8194, -17.8439) (-3.817, -17.8561) (-3.8145, -17.8683) (-3.8121, -17.8806) (-3.8096, -17.8929) (-3.8071, -17.9053) (-3.8046, -17.9176) (-3.8021, -17.93) (-3.7995, -17.9424) (-3.797, -17.9549) (-3.7943, -17.9674) (-3.7917, -17.9799) (-3.7891, -17.9924) (-3.7864, -18.005) (-3.7837, -18.0176) (-3.781, -18.0302) (-3.7782, -18.0429) (-3.7755, -18.0556) (-3.7727, -18.0683) (-3.7699, -18.081) (-3.767, -18.0938) (-3.7642, -18.1066) (-3.7613, -18.1194) (-3.7584, -18.1323) (-3.7555, -18.1451) (-3.7525, -18.158) (-3.7496, -18.171) (-3.7466, -18.1839) (-3.7435, -18.1969) (-3.7405, -18.2099) (-3.7374, -18.223) (-3.7343, -18.236) (-3.7312, -18.2491) (-3.7287, -18.2596) (-3.7268, -18.2675) (-3.7256, -18.2728) (-3.7249, -18.2754) knots 0 0 0 0 0 0 0.00416667 0.00833333 0.0125 0.01666667 0.02083333 0.025 0.02916667 0.03333333 0.0375 0.04166667 0.04583333 0.05 0.05416667 0.05833333 0.0625 0.06666667 0.07083333 0.075 0.07916667 0.08333333 0.0875 0.09166667 0.09583333 0.1 0.10416667 0.10833333 0.1125 0.11666667 0.12083333 0.125 0.12916667 0.13333333 0.1375 0.14166667 0.14583333 0.15 0.15416667 0.15833333 0.1625 0.16666667 0.17083333 0.175 0.17916667 0.18333333 0.1875 0.19166667 0.19583333 0.2 0.20416667 0.20833333 0.2125 0.21666667 0.22083333 0.225 0.22916667 0.23333333 0.2375 0.24166667 0.24583333 0.25 0.25416667 0.25833333 0.2625 0.26666667 0.27083333 0.275 0.27916667 0.28333333 0.2875 0.29166667 0.29583333 0.3 0.30416667 0.30833333 0.3125 0.31666667 0.32083333 0.325 0.32916667 0.33333333 0.3375 0.34166667 0.34583333 0.35 0.35416667 0.35833333 0.3625 0.36666667 0.37083333 0.375 0.37916667 0.38333333 0.3875 0.39166667 0.39583333 0.4 0.40416667 0.40833333 0.4125 0.41666667 0.42083333 0.425 0.42916667 0.43333333 0.4375 0.44166667 0.44583333 0.45 0.45416667 0.45833333 0.4625 0.46666667 0.47083333 0.475 0.47916667 0.48333333 0.4875 0.49166667 0.49583333 0.5 0.50416667 0.50833333 0.5125 0.51666667 0.52083333 0.525 0.52916667 0.53333333 0.5375 0.54166667 0.54583333 0.55 0.55416667 0.55833333 0.5625 0.56666667 0.57083333 0.575 0.57916667 0.58333333 0.5875 0.59166667 0.59583333 0.6 0.60416667 0.60833333 0.6125 0.61666667 0.62083333 0.625 0.62916667 0.63333333 0.6375 0.64166667 0.64583333 0.65 0.65416667 0.65833333 0.6625 0.66666667 0.67083333 0.675 0.67916667 0.68333333 0.6875 0.69166667 0.69583333 0.7 0.70416667 0.70833333 0.7125 0.71666667 0.72083333 0.725 0.72916667 0.73333333 0.7375 0.74166667 0.74583333 0.75 0.75416667 0.75833333 0.7625 0.76666667 0.77083333 0.775 0.77916667 0.78333333 0.7875 0.79166667 0.79583333 0.8 0.80416667 0.80833333 0.8125 0.81666667 0.82083333 0.825 0.82916667 0.83333333 0.8375 0.84166667 0.84583333 0.85 0.85416667 0.85833333 0.8625 0.86666667 0.87083333 0.875 0.87916667 0.88333333 0.8875 0.89166667 0.89583333 0.9 0.90416667 0.90833333 0.9125 0.91666667 0.92083333 0.925 0.92916667 0.93333333 0.9375 0.94166667 0.94583333 0.95 0.95416667 0.95833333 0.9625 0.96666667 0.97083333 0.975 0.97916667 0.98333333 0.9875 0.99166667 0.99583333 1 1 1 1 1 1
  arc A37 (-3.7249, -18.2754) -> (-2.755, -18.3773) centre (0, 12.5) ccw
  spline S37 degree 5 poles (-2.755, -18.3773) (-2.7539, -18.3749) (-2.7515, -18.37) (-2.748, -18.3627) (-2.7434, -18.353) (-2.7376, -18.3408) (-2.7319, -18.3287) (-2.7262, -18.3165) (-2.7205, -18.3044) (-2.7149, -18.2924) (-2.7092, -18.2803) (-2.7036, -18.2683) (-2.6981, -18.2563) (-2.6925, -18.2443) (-2.687, -18.2323) (-2.6815, -18.2204) (-2.6761, -18.2085) (-2.6707, -18.1966) (-2.6653, -18.1847) (-2.6599, -18.1728) (-2.6545, -18.161) (-2.6492, -18.1492) (-2.6439, -18.1374) (-2.6387, -18.1256) (-2.6335, -18.1139) (-2.6283, -18.1022) (-2.6231, -18.0905) (-2.6179, -18.0788) (-2.6128, -18.0672) (-2.6077, -18.0555) (-2.6027, -18.0439) (-2.5977, -18.0324) (-2.5927, -18.0208) (-2.5877, -18.0093) (-2.5827, -17.9978) (-2.5778, -17.9863) (-2.5729, -17.9749) (-2.5681, -17.9634) (-2.5632, -17.952) (-2.5584, -17.9407) (-2.5537, -17.9293) (-2.5489, -17.918) (-2.5442, -17.9067) (-2.5395, -17.8954) (-2.5348, -17.8841) (-2.5302, -17.8729) (-2.5256, -17.8617) (-2.521, -17.8506) (-2.5165, -17.8394) (-2.5119, -17.8283) (-2.5074, -17.8172) (-2.503, -17.8061) (-2.4985, -17.7951) (-2.4941, -17.7841) (-2.4897, -17.7731) (-2.4854, -17.7621) (-2.481, -17.7512) (-2.4767, -17.7403) (-2.4725, -17.7294) (-2.4682, -17.7186) (-2.464, -17.7078) (-2.4598, -17.697) (-2.4557, -17.6862) (-2.4515, -17.6755) (-2.4474, -17.6648) (-2.4433, -17.6541) (-2.4393, -17.6435) (-2.4353, -17.6329) (-2.4313, -17.6223) (-2.4273, -17.6118) (-2.4234, -17.6012) (-2.4194, -17.5907) (-2.4156, -17.5803) (-2.4117, -17.5699) (-2.4079, -17.5595) (-2.4041, -17.5491) (-2.4003, -17.5388) (-2.3965, -17.5284) (-2.3928, -17.5182) (-2.3891, -17.5079) (-2.3855, -17.4977) (-2.3818, -17.4875) (-2.3782, -17.4774) (-2.3746, -17.4673) (-2.3711, -17.4572) (-2.3675, -17.4471) (-2.364, -17.4371) (-2.3606, -17.4271) (-2.3571, -17.4172) (-2.3537, -17.4073) (-2.3503, -17.3974) (-2.3469, -17.3875) (-2.3436, -17.3777) (-2.3403, -17.368) (-2.337, -17.3582) (-2.3337, -17.3485) (-2.3305, -17.3388) (-2.3273, -17.3292) (-2.3241, -17.3196) (-2.321, -17.31) (-2.3178, -17.3005) (-2.3147, -17.291) (-2.3117, -17.2815) (-2.3086, -17.2721) (-2.3056, -17.2627) (-2.3026, -17.2534) (-2.2996, -17.2441) (-2.2967, -17.2348) (-2.2938, -17.2255) (-2.2909, -17.2163) (-2.288, -17.2072) (-2.2852, -17.1981) (-2.2824, -17.189) (-2.2796, -17.1799) (-2.2769, -17.1709) (-2.2741, -17.1619) (-2.2714, -17.153) (-2.2688, -17.1441) (-2.2661, -17.1353) (-2.2635, -17.1265) (-2.2609, -17.1177) (-2.2583, -17.109) (-2.2558, -17.1003) (-2.2533, -17.0917) (-2.2508, -17.083) (-2.2483, -17.0745) (-2.2458, -17.066) (-2.2434, -17.0575) (-2.241, -17.0491) (-2.2387, -17.0407) (-2.2363, -17.0323) (-2.234, -17.024) (-2.2317, -17.0158) (-2.2295, -17.0075) (-2.2272, -16.9994) (-2.225, -16.9912) (-2.2228, -16.9832) (-2.2207, -16.9751) (-2.2185, -16.9671) (-2.2164, -16.9592) (-2.2143, -16.9513) (-2.2123, -16.9434) (-2.2102, -16.9356) (-2.2082, -16.9279) (-2.2062, -16.9202) (-2.2043, -16.9125) (-2.2023, -16.9049) (-2.2004, -16.8973) (-2.1985, -16.8898) (-2.1967, -16.8823) (-2.1948, -16.8749) (-2.193, -16.8675) (-2.1912, -16.8602) (-2.1895, -16.8529) (-2.1877, -16.8457) (-2.186, -16.8386) (-2.1843, -16.8314) (-2.1827, -16.8244) (-2.181, -16.8174) (-2.1794, -16.8104) (-2.1778, -16.8035) (-2.1762, -16.7967) (-2.1747, -16.7899) (-2.1731, -16.7831) (-2.1716, -16.7764) (-2.1702, -16.7698) (-2.1687, -16.7632) (-2.1673, -16.7567) (-2.1659, -16.7502) (-2.1645, -16.7438) (-2.1631, -16.7374) (-2.1618, -16.7311) (-2.1605, -16.7249) (-2.1592, -16.7187) (-2.1579, -16.7126) (-2.1567, -16.7065) (-2.1554, -16.7005) (-2.1542, -16.6946) (-2.153, -16.6887) (-2.1519, -16.6829) (-2.1507, -16.6771) (-2.1496, -16.6714) (-2.1485, -16.6658) (-2.1475, -16.6602) (-2.1464, -16.6547) (-2.1454, -16.6493) (-2.1444, -16.6439) (-2.1434, -16.6386) (-2.1424, -16.6334) (-2.1415, -16.6282) (-2.1406, -16.6231) (-2.1397, -16.618) (-2.1388, -16.6131) (-2.138, -16.6081) (-2.1371, -16.6033) (-2.1363, -16.5985) (-2.1355, -16.5938) (-2.1347, -16.5892) (-2.134, -16.5847) (-2.1332, -16.5802) (-2.1325, -16.5758) (-2.1318, -16.5714) (-2.1312, -16.5672) (-2.1305, -16.563) (-2.1299, -16.5589) (-2.1292, -16.5549) (-2.1286, -16.5509) (-2.1281, -16.547) (-2.1275, -16.5432) (-2.127, -16.5395) (-2.1264, -16.5359) (-2.1259, -16.5323) (-2.1254, -16.5289) (-2.125, -16.5255) (-2.1245, -16.5222) (-2.1241, -16.5189) (-2.1237, -16.5158) (-2.1233, -16.5128) (-2.1229, -16.5098) (-2.1225, -16.5069) (-2.1222, -16.5041) (-2.1219, -16.5015) (-2.1215, -16.4989) (-2.1212, -16.4963) (-2.121, -16.4939) (-2.1207, -16.4916) (-2.1204, -16.4894) (-2.1202, -16.4873) (-2.12, -16.4852) (-2.1198, -16.4833) (-2.1196, -16.4815) (-2.1194, -16.4798) (-2.1192, -16.4781) (-2.1191, -16.4766) (-2.1189, -16.4752) (-2.1188, -16.4739) (-2.1187, -16.4727) (-2.1186, -16.4716) (-2.1185, -16.4706) (-2.1184, -16.4698) (-2.1184, -16.469) (-2.1183, -16.4685) (-2.1183, -16.4682) (-2.1183, -16.468) (-2.1183, -16.4679) knots -1 -1 -1 -1 -1 -1 -0.99583333 -0.99166667 -0.9875 -0.98333333 -0.97916667 -0.975 -0.97083333 -0.96666667 -0.9625 -0.95833333 -0.95416667 -0.95 -0.94583333 -0.94166667 -0.9375 -0.93333333 -0.92916667 -0.925 -0.92083333 -0.91666667 -0.9125 -0.90833333 -0.90416667 -0.9 -0.89583333 -0.89166667 -0.8875 -0.88333333 -0.87916667 -0.875 -0.87083333 -0.86666667 -0.8625 -0.85833333 -0.85416667 -0.85 -0.84583333 -0.84166667 -0.8375 -0.83333333 -0.82916667 -0.825 -0.82083333 -0.81666667 -0.8125 -0.80833333 -0.80416667 -0.8 -0.79583333 -0.79166667 -0.7875 -0.78333333 -0.77916667 -0.775 -0.77083333 -0.76666667 -0.7625 -0.75833333 -0.75416667 -0.75 -0.74583333 -0.74166667 -0.7375 -0.73333333 -0.72916667 -0.725 -0.72083333 -0.71666667 -0.7125 -0.70833333 -0.70416667 -0.7 -0.69583333 -0.69166667 -0.6875 -0.68333333 -0.67916667 -0.675 -0.67083333 -0.66666667 -0.6625 -0.65833333 -0.65416667 -0.65 -0.64583333 -0.64166667 -0.6375 -0.63333333 -0.62916667 -0.625 -0.62083333 -0.61666667 -0.6125 -0.60833333 -0.60416667 -0.6 -0.59583333 -0.59166667 -0.5875 -0.58333333 -0.57916667 -0.575 -0.57083333 -0.56666667 -0.5625 -0.55833333 -0.55416667 -0.55 -0.54583333 -0.54166667 -0.5375 -0.53333333 -0.52916667 -0.525 -0.52083333 -0.51666667 -0.5125 -0.50833333 -0.50416667 -0.5 -0.49583333 -0.49166667 -0.4875 -0.48333333 -0.47916667 -0.475 -0.47083333 -0.46666667 -0.4625 -0.45833333 -0.45416667 -0.45 -0.44583333 -0.44166667 -0.4375 -0.43333333 -0.42916667 -0.425 -0.42083333 -0.41666667 -0.4125 -0.40833333 -0.40416667 -0.4 -0.39583333 -0.39166667 -0.3875 -0.38333333 -0.37916667 -0.375 -0.37083333 -0.36666667 -0.3625 -0.35833333 -0.35416667 -0.35 -0.34583333 -0.34166667 -0.3375 -0.33333333 -0.32916667 -0.325 -0.32083333 -0.31666667 -0.3125 -0.30833333 -0.30416667 -0.3 -0.29583333 -0.29166667 -0.2875 -0.28333333 -0.27916667 -0.275 -0.27083333 -0.26666667 -0.2625 -0.25833333 -0.25416667 -0.25 -0.24583333 -0.24166667 -0.2375 -0.23333333 -0.22916667 -0.225 -0.22083333 -0.21666667 -0.2125 -0.20833333 -0.20416667 -0.2 -0.19583333 -0.19166667 -0.1875 -0.18333333 -0.17916667 -0.175 -0.17083333 -0.16666667 -0.1625 -0.15833333 -0.15416667 -0.15 -0.14583333 -0.14166667 -0.1375 -0.13333333 -0.12916667 -0.125 -0.12083333 -0.11666667 -0.1125 -0.10833333 -0.10416667 -0.1 -0.09583333 -0.09166667 -0.0875 -0.08333333 -0.07916667 -0.075 -0.07083333 -0.06666667 -0.0625 -0.05833333 -0.05416667 -0.05 -0.04583333 -0.04166667 -0.0375 -0.03333333 -0.02916667 -0.025 -0.02083333 -0.01666667 -0.0125 -0.00833333 -0.00416667 0 0 0 0 0 0
  line L75 (-2.1183, -16.4679) -> (-2.1182, -16.4671)
  line L76 (-2.1182, -16.4671) -> (-2.0967, -16.1734)
  arc A38 (-2.0967, -16.1734) -> (-0.9119, -16.2355) centre (0, 12.5) ccw
  line L77 (-0.9119, -16.2355) -> (-0.9213, -16.5298)
  line L78 (-0.9213, -16.5298) -> (-0.9213, -16.5307)